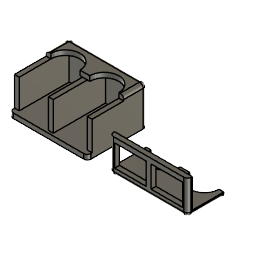
Button rig 3 (Autodesk Fusion 360 design; units mm, degrees)
part number: 2026-01-31-14-33-28-622
Autodesk Fusion 360 part; units mm, degrees
sketch "Sketch1" plane through (0, 0, 0) normal (0, 0, 1) x (1, 0, 0)
  line L0 (16, 12.25) -> (-16, 12.25)
  line L1 (-16, 12.25) -> (-16, -12.25)
  line L2 (-16, -12.25) -> (16, -12.25)
  line L3 (16, -12.25) -> (16, 12.25)
  line L4 (16, 12.25) -> (-16, -12.25) construction
  line L5 (-16, 12.25) -> (16, -12.25) construction
  dimension "d1" = 32
  dimension "d2" = 24.5
  constraint horizontal L0
  constraint perpendicular L0 L1
  constraint parallel L0 L2
  constraint parallel L1 L3
  constraint coincident L4 origin
  constraint coincident L5 origin
  measures "d1" distance of L1.end L2.end
  measures "d2" distance of L0.end L1.end
extrude "Extrude1" add sketch "Sketch1" along normal blind 2 makes body 1
sketch "Sketch3" plane through (0, 0, 2) normal (0, 0, 1) x (-1, 0, 0)
  line L0 (-16, 12.25) -> (-16, -12.25)
  line L1 (-16, -12.25) -> (16, -12.25)
  line L2 (16, -12.25) -> (16, 12.25)
  line L3 (16, 12.25) -> (-16, 12.25)
  line L4 (16, -12.25) -> (14, -12.25)
  line L5 (14, -12.25) -> (14, 10.25)
  line L6 (14, 10.25) -> (16, 10.25)
  line L7 (16, 10.25) -> (16, -12.25)
  line L8 (16, -12.25) -> (-16, -12.25)
  line L9 (-16, -12.25) -> (-16, -10.25)
  line L10 (-16, -10.25) -> (16, -10.25)
  line L11 (16, -10.25) -> (16, -12.25)
  line L12 (-16, -12.25) -> (-14, -12.25)
  line L13 (-14, -12.25) -> (-14, 10.25)
  line L14 (-14, 10.25) -> (-16, 10.25)
  line L15 (-16, 10.25) -> (-16, -12.25)
  line L16 (1, -11.25) -> (-1, -11.25)
  line L17 (-1, -11.25) -> (-1, 11.25)
  line L18 (-1, 11.25) -> (1, 11.25)
  line L19 (1, 11.25) -> (1, -11.25)
  line L20 (1, -11.25) -> (-1, 11.25) construction
  line L21 (-1, -11.25) -> (1, 11.25) construction
  dimension "d5" = 2
  dimension "d6" = 2
  dimension "d7" = 2
  dimension "d8" = 20.5
  dimension "d9" = 20.5
  dimension "d25" = 2
  dimension "d40" = 21.5
  constraint horizontal L4
  constraint vertical L5
  constraint horizontal L6
  constraint vertical L7
  constraint coincident L1.end L2.start
  constraint horizontal L8
  constraint vertical L9
  constraint horizontal L10
  constraint vertical L11
  constraint horizontal L12
  constraint vertical L13
  constraint horizontal L14
  constraint vertical L15
  constraint coincident L0.end L1.start
  constraint horizontal L16
  constraint perpendicular L16 L17
  constraint parallel L16 L18
  constraint parallel L17 L19
  constraint coincident L20 origin
  constraint coincident L21 origin
  measures "d5" distance of L1.end L4.end
  measures "d6" distance of L1.end L10.end
  measures "d7" distance of L0.end L12.end
  measures "d8" distance of L6 L10
  measures "d9" distance of L10 L14
  measures "d25" distance of L17.end L18.end
  measures "d40" distance of L10 L18
extrude "Extrude2" add sketch "Sketch3" along normal blind 12 contours L0 L10 L13 L14 L15 | L0 L1 L8 L9 L10 L12 L13 L15 | L2 L5 L6 L7 L10 | L1 L5 L8 L10 L13 L16 L17 L19 | L1 L2 L4 L5 L7 L8 L10 L11 | L10 L17 L18 L19 | L10 L16 L17 L19 bodies 1
sketch "Sketch4" plane through (0, 0, 14) normal (0, 0, 1) x (-1, 0, 0)
  line L0 (-14, -10.25) -> (-14, 10.25)
  line L1 (-14, 10.25) -> (-16, 10.25)
  line L2 (-16, 10.25) -> (-16, -12.25)
  line L3 (-16, -12.25) -> (16, -12.25)
  line L4 (16, -12.25) -> (16, 10.25)
  line L5 (16, 10.25) -> (14, 10.25)
  line L6 (14, 10.25) -> (14, -10.25)
  line L7 (14, -10.25) -> (1, -10.25)
  line L8 (16, -12.25) -> (-16, -12.25)
  line L9 (-16, -12.25) -> (-16, -2.75)
  line L10 (-16, -2.75) -> (16, -2.75)
  line L11 (16, -2.75) -> (16, -12.25)
  line L12 (1, -10.25) -> (1, 11.25)
  line L13 (1, 11.25) -> (-1, 11.25)
  line L14 (-1, 11.25) -> (-1, -10.25)
  line L15 (-1, -10.25) -> (-14, -10.25)
  circle A0 centre (8, -2.75) radius 6
  circle A1 centre (-8, -2.75) radius 6
  point P0 (8, -2.75)
  point P1 (-8, -2.75)
  dimension "d12" = 9.5
  dimension "d26" = 9.5
  dimension "d27" = 8
  dimension "d28" = 12
  dimension "d29" = 9.5
  dimension "d30" = 8
  dimension "d31" = 12
  constraint horizontal L8
  constraint vertical L9
  constraint horizontal L10
  constraint vertical L11
  constraint coincident L3.end L4.start
  constraint coincident P0 A0.centre
  constraint coincident P1 A1.centre
  measures "d12" distance of L3.end L10.end
  measures "d26" distance of L8 P0
  measures "d27" distance of L11 P0
  measures "d28" diameter of A0
  measures "d29" distance of L8 P1
  measures "d30" distance of L9.end P1
  measures "d31" diameter of A1
extrude "Extrude3" add sketch "Sketch4" along normal blind 2 contours L0 L2 L3 L4 L6 L7 L8 L9 L10 L11 L12 L14 L15 | L0 L10 L14 L15 A1 | L6 L7 L10 L12 A0 bodies 1
sketch "Sketch6" plane through (0, 0, 0) normal (0, 0, 1) x (1, 0, 0)
  line L0 (25, 3) -> (41, 3)
  line L1 (41, 3) -> (41, -12)
  line L2 (41, -12) -> (25, -12)
  line L3 (25, -12) -> (25, 3)
  circle A0 centre (33, 3) radius 6
  line L4 (57, -12) -> (57, 3)
  line L5 (41, -12) -> (57, -12)
  line L6 (57, 3) -> (41, 3)
  circle A1 centre (49, 3) radius 6
  line L7 (41, 3) -> (41, -12)
  point P0 (33, 3)
  point P1 (33, 3)
  point P2 (49, 3)
  point P3 (49, 3)
  dimension "d32" = 16
  dimension "d35" = 8
  dimension "d36" = 12
  dimension "d39" = 15
  constraint horizontal L0
  constraint vertical L1
  constraint horizontal L2
  constraint vertical L3
  constraint coincident L0 P1
  constraint coincident P1 P0
  constraint midpoint L0 P1
  constraint symmetric L0.start L1 L4.end
  constraint symmetric L0.end L1 L6.end
  constraint symmetric L2.start L1 L5.start
  constraint symmetric L2.end L1 L4.start
  constraint symmetric L1 P1 P3
  constraint symmetric L1 A0 A1
  measures "d32" distance of L0.start L0.end
  measures "d35" distance of L3 P1
  measures "d36" diameter of A0
  measures "d39" distance of L0 L2
extrude "Extrude4" add sketch "Sketch6" along normal blind 2 separate body contours L0 L1 L2 L3 A0 L7 | L1 L4 L5 L6 A1 L7 makes body 2
move_face "MoveFace1" by (-4.6593, -0.2769, -0.0747) 1 faces at (33.1495, -8.9944, 2) on bodies 2
sketch "Sketch7" plane through (0, 0, 1.9253) normal (0, 0, 1) x (-1, 0, 0)
  line L0 (-25, 12) -> (-57, 12)
  line L1 (-57, 12) -> (-57, -3)
  line L2 (-57, -3) -> (-55, -3)
  arc A0 (-43, -3) -> (-55, -3) centre (-49, -3) ccw
  line L3 (-43, -3) -> (-39, -3)
  arc A1 (-27, -3) -> (-39, -3) centre (-33, -3) ccw
  line L4 (-27, -3) -> (-25, -3)
  line L5 (-25, -3) -> (-25, 12)
  line L6 (-25, 10) -> (-57, 10)
  line L7 (-57, 10) -> (-57, 12)
  line L8 (-57, 12) -> (-25, 12)
  line L9 (-25, 12) -> (-25, 10)
  line L10 (-40, -3) -> (-42, -3)
  line L11 (-42, -3) -> (-42, 12)
  line L12 (-42, 12) -> (-40, 12)
  line L13 (-40, 12) -> (-40, -3)
  line L14 (-25, -3) -> (-27, -3)
  line L15 (-27, -3) -> (-27, 12)
  line L16 (-27, 12) -> (-25, 12)
  line L17 (-25, 12) -> (-25, -3)
  line L18 (-55, -3) -> (-57, -3)
  line L19 (-57, -3) -> (-57, 12)
  line L20 (-57, 12) -> (-55, 12)
  line L21 (-55, 12) -> (-55, -3)
  dimension "d59" = 2
  constraint horizontal L6
  constraint vertical L7
  constraint horizontal L8
  constraint vertical L9
  constraint coincident L0.end L1.start
  constraint coincident L5 L6.start
  constraint horizontal L10
  constraint vertical L11
  constraint horizontal L12
  constraint vertical L13
  constraint coincident L8 L11.end
  constraint horizontal L14
  constraint vertical L15
  constraint horizontal L16
  constraint vertical L17
  constraint coincident L8 L15.end
  constraint coincident L4.end L5.start
  constraint horizontal L18
  constraint vertical L19
  constraint horizontal L20
  constraint vertical L21
  constraint coincident L2.end A0.end
  measures "d59" distance of L6 L8
extrude "Extrude5" add sketch "Sketch7" along normal blind 1 contours L0 L6 L8 L13 L15 | L0 L6 L8 L11 L21 bodies 2
extrude "Extrude6" add sketch "Sketch7" along normal blind 12 contours L0 L5 L6 L8 L9 L15 L16 L17 | L0 L6 L8 L11 L12 L13 | L0 L1 L6 L7 L8 L19 L20 L21 bodies 2
sketch "Sketch9" plane through (0, 0, 13.9253) normal (0, 0, 1) x (-1, 0, 0)
  line L0 (-25, 12) -> (-27, 12)
  line L1 (-27, 12) -> (-27, 10)
  line L2 (-27, 10) -> (-25, 10)
  line L3 (-25, 10) -> (-25, 12)
  line L4 (-27, 10) -> (-40, 10)
  line L5 (-40, 10) -> (-40, 12)
  line L6 (-40, 12) -> (-27, 12)
  line L7 (-27, 12) -> (-27, 10)
  line L8 (-55, 12) -> (-42, 12)
  line L9 (-42, 12) -> (-42, 10)
  line L10 (-42, 10) -> (-55, 10)
  line L11 (-55, 10) -> (-55, 12)
  constraint horizontal L4
  constraint vertical L5
  constraint horizontal L6
  constraint vertical L7
  constraint coincident L1.end L2.start
  constraint horizontal L8
  constraint vertical L9
  constraint horizontal L10
  constraint vertical L11
extrude "Extrude7" add sketch "Sketch9" against normal blind 2 contours L1 L4 L5 L6 L7 | L8 L9 L10 L11 bodies 2
fillet "Fillet7" radius 1.5 5 edges at (41, -12, 0) (57, -12, 6.9627) (57, -4.5, 0) (25, -4.5, 0) (25, -12, 6.9627) on bodies 2
fillet "Fillet1" radius 1.5 7 edges at (16, 12.25, 8) (0, 12.25, 16) (16, 7.5, 16) (-16, 7.5, 16) (-16, 12.25, 8) (-16, -12.25, 1) (16, -12.25, 1) on bodies 1
